Protege connecteur (Autodesk Fusion 360 design; units mm, degrees)
Autodesk Fusion 360 part; units mm, degrees
note: some values were not read from the file. Set by a fixed rule: which sketch regions a step uses.
sketch "Sketch1" plane through (0, 0, 0) normal (0, 1, 0) x (1, 0, 0)
  line L0 (0, -19) -> (2.5, -19)
  line L1 (2.5, -17) -> (2.5, 0)
  line L2 (2.5, 0) -> (0, 0)
  line L3 (0, 0) -> (0, -19)
  line L4 (10, -0.0285) -> (11, -0.0285)
  line L5 (11, -0.0285) -> (11, -16.0285)
  line L6 (11, -16.0285) -> (10, -16.0285) construction
  line L7 (10, -16.0285) -> (10, -0.0285)
  line L8 (2.5, -17) -> (-5, -17) construction
  line L9 (2.5, -17) -> (2.5, -19) construction
  arc A0 (2.5, -17) -> (10, -16.0285) centre (2.5, 12.4344) ccw
  arc A1 (2.5, -19) -> (11, -16.0285) centre (2.5, -5.3573) ccw
  dimension "d1" = 2.5
  dimension "d2" = 1
  dimension "d5" = 19
  dimension "d6" = 11
  dimension "d8" = 17
  dimension "d9" = 16
  constraint horizontal L0
  constraint vertical L1
  constraint horizontal L2
  constraint vertical L3
  constraint horizontal L4
  constraint vertical L5
  constraint horizontal L6
  constraint vertical L7
  constraint perpendicular L3 L8
  constraint perpendicular L8 L9
  constraint tangent L8 A0
  constraint tangent L0 A1
  measures "d1" distance of L1.end L2.end
  measures "d2" distance of L5.end L6.end
  measures "d5" distance of L0 L2
  measures "d6" distance of L3 L5
  measures "d8" distance of L1.end L1.start
  measures "d9" distance of L4.end L6
revolve "Revolve1" add sketch "Sketch1" angle 360 about axis through (0, 0, -3.23) along (0, 0, 1)
